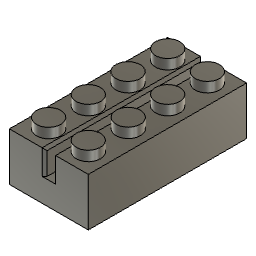
Robo_Robin_Fuß v4 (Autodesk Fusion 360 design; units mm, degrees)
Autodesk Fusion 360 part; units mm, degrees
sketch "Skizze1" plane through (0, 0, 0) normal (0, 0, 1) x (1, 0, 0)
  line L0 (0, 0) -> (15.9, 0)
  line L1 (15.9, 0) -> (15.9, 31.9)
  line L2 (15.9, 31.9) -> (0, 31.9)
  line L3 (0, 31.9) -> (0, 0)
  circle A0 centre (7.95, 15.95) radius 3.2
  circle A1 centre (7.95, 15.95) radius 2.2
  circle A2 centre (8, 24) radius 3.2
  circle A3 centre (8, 24) radius 2.2
  line L4 (14.4, 30.4) -> (1.5, 30.4)
  line L5 (1.5, 30.4) -> (1.5, 1.5)
  line L6 (1.5, 1.5) -> (14.4, 1.5)
  line L7 (14.4, 1.5) -> (14.4, 30.4)
  circle A4 centre (8, 7.9) radius 3.2
  circle A5 centre (8, 7.9) radius 2.2
  dimension "d1" = 15.9
  dimension "d2" = 31.9
  dimension "d3" = 6.4
  dimension "d4" = -1
  dimension "d5" = 15.9
  dimension "d6" = 7.95
  dimension "d7" = 6.4
  dimension "d8" = -1
  dimension "d10" = -1.5
  dimension "d11" = 6.4
  dimension "d12" = 6.4
  dimension "d13" = -1
  dimension "d14" = 6.4
  constraint horizontal L0
  constraint vertical L1
  constraint horizontal L2
  constraint vertical L3
  constraint coincident L0.start L3.end
  measures "d1" distance of L1.end L2.end
  measures "d2" distance of L0.end L1.end
  measures "d3" diameter of A0
  measures "d5" distance of L0.start L0.end
  measures "d6" distance of L1 A0.centre
  measures "d7" diameter of A2
  measures "d11" distance of A2.centre L4
  measures "d12" diameter of A4
  measures "d14" distance of L6 A4.centre
extrude "Extrusion1" add sketch "Skizze1" along normal blind 9.7 makes body 1 at (11.196, 7.7405, 6.4667) makes body 2 at (11.146, 15.7905, 6.4667) makes body 3 at (0, 21.2667, 6.4667) makes body 4 at (11.196, 23.8405, 6.4667)
sketch "Skizze2" plane through (0, 0, 9.7) normal (0, 0, 1) x (-1, 0, 0)
  line L0 (-14.4, -30.4) -> (-14.4, -1.5)
  line L1 (-14.4, -1.5) -> (-1.5, -1.5)
  line L2 (-1.5, -1.5) -> (-1.5, -30.4)
  line L3 (-1.5, -30.4) -> (-14.4, -30.4)
  line L4 (0, -31.9) -> (0, 0)
  line L5 (0, 0) -> (-15.9, 0)
  line L6 (-15.9, 0) -> (-15.9, -31.9)
  line L7 (-15.9, -31.9) -> (0, -31.9)
  line L8 (0, 0) -> (-15.9, 0)
  line L9 (-15.9, 0) -> (-15.9, -31.9)
  line L10 (-15.9, -31.9) -> (0, -31.9)
  line L11 (0, -31.9) -> (0, 0)
  constraint horizontal L8
  constraint vertical L9
  constraint horizontal L10
  constraint vertical L11
  constraint coincident L6.end L7.start
  constraint coincident L4.end L5.start
extrude "Extrusion2" add sketch "Skizze2" against normal blind 1.5 contours L0 L1 L2 L3 | L4 L5 L6 L7 L8 L9 L10 L11 bodies 1 2 3 4
sketch "Skizze3" plane through (0, 0, 9.7) normal (0, 0, 1) x (-1, 0, 0)
  line L0 (0, -31.9) -> (0, 0)
  line L1 (0, 0) -> (-15.9, 0)
  line L2 (-15.9, 0) -> (-15.9, -31.9)
  line L3 (-15.9, -31.9) -> (0, -31.9)
  circle A0 centre (-3.95, -27.95) radius 2.45
  circle A1 centre (-3.95, -19.95) radius 2.45
  circle A2 centre (-3.95, -11.95) radius 2.45
  circle A3 centre (-3.95, -3.95) radius 2.45
  circle A4 centre (-11.95, -3.95) radius 2.45
  circle A5 centre (-11.95, -12) radius 2.45
  circle A6 centre (-11.95, -19.95) radius 2.45
  circle A7 centre (-11.95, -27.95) radius 2.45
  dimension "d19" = 4.9
  dimension "d20" = 4.9
  dimension "d21" = 4.9
  dimension "d22" = 4.9
  dimension "d23" = 4.9
  dimension "d24" = 4.9
  dimension "d25" = 4.9
  dimension "d26" = 4.9
  dimension "d27" = 8
  dimension "d28" = 8
  dimension "d29" = 8
  dimension "d30" = 8
  dimension "d31" = 15.9
  dimension "d32" = 3.95
  dimension "d33" = 3.95
  dimension "d34" = 3.95
  dimension "d35" = 3.95
  dimension "d36" = 8
  dimension "d37" = 8
  dimension "d38" = 8
  dimension "d39" = 31.9
  dimension "d40" = 3.95
  dimension "d41" = 3.95
  measures "d19" diameter of A0
  measures "d20" diameter of A1
  measures "d21" diameter of A2
  measures "d22" diameter of A3
  measures "d23" diameter of A4
  measures "d24" diameter of A5
  measures "d25" diameter of A6
  measures "d26" diameter of A7
  measures "d27" distance of A0.centre A7.centre
  measures "d28" distance of A1.centre A6.centre
  measures "d29" horizontal distance of A2.centre A5.centre
  measures "d30" distance of A3.centre A4.centre
  measures "d31" distance of L0.end L1.end
  measures "d32" distance of L2 A7.centre
  measures "d33" distance of L2 A6.centre
  measures "d34" distance of L2 A5.centre
  measures "d35" distance of L2 A4.centre
  measures "d36" distance of A0.centre A1.centre
  measures "d37" distance of A1.centre A2.centre
  measures "d38" distance of A2.centre A3.centre
  measures "d39" distance of L0.start L0.end
  measures "d40" distance of L3 A0.centre
  measures "d41" distance of L1 A4.centre
extrude "Extrusion3" add sketch "Skizze3" along normal blind 2 contours A0 | A1 | A2 | A3 | A4 | A5 | A6 | A7 bodies 1
sketch "Skizze4" plane through (0, 0, 9.7) normal (0, 0, 1) x (-1, 0, 0)
  circle A0 centre (-11.95, -19.95) radius 2.45
  circle A1 centre (-3.95, -11.95) radius 2.45
  circle A2 centre (-3.95, -3.95) radius 2.45
  circle A3 centre (-3.95, -19.95) radius 2.45
  circle A4 centre (-11.95, -27.95) radius 2.45
  circle A5 centre (-11.95, -12) radius 2.45
  circle A6 centre (-11.95, -3.95) radius 2.45
  circle A7 centre (-3.95, -27.95) radius 2.45
  line L0 (0, -31.9) -> (0, 0)
  line L1 (0, 0) -> (-15.9, 0)
  line L2 (-15.9, 0) -> (-15.9, -31.9)
  line L3 (-15.9, -31.9) -> (0, -31.9)
  line L4 (-7.125, -31.9) -> (-8.775, -31.9)
  line L5 (-8.775, -31.9) -> (-8.775, 4.1)
  line L6 (-8.775, 4.1) -> (-7.125, 4.1)
  line L7 (-7.125, 4.1) -> (-7.125, -31.9)
  dimension "d44" = 1.65
  constraint horizontal L4
  constraint vertical L5
  constraint horizontal L6
  constraint vertical L7
  constraint midpoint L3 L4
  measures "d44" distance of L4.start L4.end
extrude "Extrusion4" cut sketch "Skizze4" against normal blind 5 contours L1 L3 L4 L5 L7 bodies 1
sketch "Skizze5" plane through (0, 0, 9.7) normal (0, 0, 1) x (-1, 0, 0)
  line L0 (-7.125, 0) -> (-7.125, -31.9)
  line L1 (-7.125, -31.9) -> (0, -31.9)
  line L2 (0, -31.9) -> (0, 0)
  line L3 (0, 0) -> (-7.125, 0)
  circle A0 centre (-3.95, -27.95) radius 2.45
  circle A1 centre (-3.95, -19.95) radius 2.45
  circle A2 centre (-3.95, -3.95) radius 2.45
  circle A3 centre (-3.95, -11.95) radius 2.45
  line L4 (-7.125, -31.9) -> (-8.775, -31.9)
  line L5 (-8.775, -31.9) -> (-8.775, 0.6)
  line L6 (-8.775, 0.6) -> (-7.125, 0.6)
  line L7 (-7.125, 0.6) -> (-7.125, -31.9)
  line L8 (-6.125, -31.9) -> (-9.775, -31.9)
  line L9 (-9.775, -31.9) -> (-9.775, 0)
  line L10 (-9.775, 0) -> (-6.125, 0)
  line L11 (-6.125, 0) -> (-6.125, -31.9)
  line L12 (-8.775, 0) -> (-7.125, 0)
  dimension "d47" = 1.65
  dimension "d48" = 3.65
  constraint horizontal L4
  constraint vertical L5
  constraint horizontal L6
  constraint vertical L7
  constraint coincident L0.end L1.start
  constraint horizontal L8
  constraint vertical L9
  constraint horizontal L10
  constraint vertical L11
  constraint coincident L1 L8.start
  constraint midpoint L10 L12
  measures "d47" distance of L5.end L6.end
  measures "d48" distance of L9.end L10.end
extrude "Extrusion5" add sketch "Skizze5" against normal blind 5 contours L0 L1 L3 A0 A1 A2 A3 L7 L8 L10 L11 | L5 L8 L9 L10 | A2 L11 | A0 L11 | A3 L11 | A1 L11 picked at (-6.1695, -3.6764) picked at (-6.1695, -28.2236) picked at (-6.1695, -11.6764) picked at (-6.1695, -20.2236) bodies 1
extrude "Extrusion6" add 6 faces at (9.8249, 7.5448, 8.2) (9.8288, 16.2653, 8.2) (9.8249, 23.6448, 8.2) (6.0783, 8.1942, 8.2) (6.0712, 16.2653, 8.2) (6.0783, 23.7058, 8.2) along direction (0, 0, -1) blind 4.5 on bodies 1 bodies 1
sketch "Skizze6" plane through (0, 0, 4.7) normal (0, 0, -1) x (1, 0, 0)
  line L0 (7.125, -1.5) -> (6.125, -1.5)
  line L1 (6.125, -1.5) -> (6.125, -5.3069)
  arc A0 (7.125, -4.822) -> (6.125, -5.3069) centre (8, -7.9) ccw
  line L2 (7.125, -4.822) -> (7.125, -1.5)
  line L3 (6.125, -1.5) -> (9.775, -1.5)
  line L4 (9.775, -1.5) -> (9.775, -30.4)
  line L5 (9.775, -30.4) -> (6.125, -30.4)
  line L6 (6.125, -30.4) -> (6.125, -1.5)
  dimension "d53" = 3.65
  dimension "d54" = 28.9
  constraint horizontal L3
  constraint vertical L4
  constraint horizontal L5
  constraint vertical L6
  constraint coincident L0.end L1.start
  measures "d53" distance of L4.end L5.end
  measures "d54" distance of L3.end L4.end
extrude "Extrusion7" add sketch "Skizze6" along normal blind 1 bodies 1
move_face "Flächen versetzen1" offset -0.025 1 faces at (7.125, 10.6333, 8.0333) on bodies 1
move_face "Flächen versetzen2" offset -0.025 1 faces at (8.775, 21.2667, 8.0333) on bodies 1
chamfer "Fase1" distance 0.5 angle 45 6 edges at (7.1, 0, 7.2) (8.8, 0, 7.2) (7.1, 15.95, 9.7) (8.8, 15.95, 9.7) (8.8, 31.9, 7.2) (7.1, 31.9, 7.2) on bodies 1
equation "d6 = ( 15.9 / 2 ) * 1 mm"
equation "d27 = 4.9 mm + 3.1 mm"
equation "d32 = 1.5 mm + 2.45 mm"
equation "d36 = 4.9 mm + 3.1 mm"
